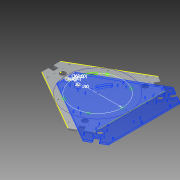
# Autodesk Inventor part: build deck
Saved by Autodesk Inventor 2015 SP1 (Build 190203100, 203)
## iProperties
Created: 2015-01-31
Part Number: build deck
Material: Generic
Document SubType Name: Modeling
Designer: Joseph
Density: 1 g/cm^3
Appearance: Clear
Author: Joseph
Autodesk Inventor part; units mm, degrees
ref_plane "YZ Plane" through (0, 0, 0) normal (1, 0, 0) x (0, 1, 0)
ref_plane "XZ Plane" through (0, 0, 0) normal (0, 1, 0) x (-1, 0, 0)
ref_plane "XY Plane" through (0, 0, 0) normal (0, 0, 1) x (1, 0, 0)
sketch "Sketch1" plane through (0, 0, 0) normal (0, 0, 1) x (1, 0, 0)
  line L0 (-22.3671, -44.8758) -> (185.479, -164.8758)
  line L1 (263.2049, -120.0008) -> (263.2049, 119.9992)
  line L2 (263.2049, 138.0318) -> (240.8188, 150.9564)
  line L3 (201.0957, -173.8921) -> (223.4817, -160.9675)
  line L4 (-37.9837, -10.0104) -> (-37.9837, -35.8596)
  line L5 (263.2049, 138.0318) -> (263.2049, -138.0333)
  line L6 (201.0957, -173.8921) -> (-37.9837, -35.8596)
  line L7 (-37.9837, 9.9896) -> (-17.9837, 9.9896)
  line L8 (-17.9837, 9.9896) -> (-17.9837, -10.0104)
  line L9 (-17.9837, -10.0104) -> (-37.9837, -10.0104)
  line L10 (-37.9837, -35.8596) -> (-37.9837, -10.0104)
  line L11 (-37.9837, 9.9896) -> (-37.9837, 35.8388)
  line L12 (223.49, -160.9627) -> (213.49, -143.6422)
  line L13 (213.49, -143.6422) -> (230.8105, -133.6422)
  line L14 (230.8105, -133.6422) -> (240.8105, -150.9627)
  line L15 (263.2049, -138.0333) -> (240.8105, -150.9627)
  line L16 (223.49, -160.9627) -> (201.0957, -173.8921)
  line L17 (223.5235, 160.9901) -> (213.4873, 143.6905)
  line L18 (213.4873, 143.6905) -> (230.7869, 133.6543)
  line L19 (230.7869, 133.6543) -> (240.7869, 150.9748)
  line L20 (201.1375, 173.9147) -> (223.5235, 160.9901)
  line L21 (240.7869, 150.9748) -> (263.2049, 138.0318)
  line L22 (-37.9837, 35.8388) -> (201.1375, 173.9147)
  point P0 (0, 0)
  dimension "d0" = 20
  dimension "d1" = 20
  dimension "d2" = 20
  dimension "d3" = 20
  dimension "d4" = 20
  dimension "d5" = 20
  constraints: 46 end point, 10 perpendicular, 5 equal length, 5 vertical, 2 collinear, 2 parallel, 1 horizontal, 13 other
  measures "d0" distance of L7.start L7.end
  measures "d1" distance of L7.end L8.end
  measures "d2" distance of L12.start L12.end
  measures "d3" distance of L12.end L13.end
  measures "d4" distance of L17.start L17.end
  measures "d5" distance of L17.end L18.end
extrude "Extrusion1" add sketch "Sketch1" along normal blind 6.35
sketch "Sketch2" plane through (0, 0, 6.35) normal (0, 0, 1) x (1, 0, 0)
  line L0 (201.1375, 173.9147) -> (-37.9837, 35.8388) projected
  line L1 (-37.9837, -35.8596) -> (201.0957, -173.8921) projected
  line L2 (263.2049, -138.0333) -> (263.2049, 138.0318) projected
  line L3 (-13.2714, -20.105) -> (-13.2714, 20.0856) projected
  line L4 (237.2204, -124.5359) -> (202.4143, -144.6312) projected
  line L5 (202.4143, 144.6118) -> (237.2204, 124.5165) projected
  line L6 (-13.2714, -0.0097) -> (263.2049, -0.0008) construction
  line L7 (219.8173, 134.5641) -> (81.556, -104.8758) construction
  line L8 (219.8173, -134.5836) -> (81.5535, 104.8633) construction
  circle A0 centre (142.1099, -0.009) radius 90 construction
  line L9 (-13.2714, -21.259) -> (29.2286, -21.259) construction
  line L10 (29.2286, -21.259) -> (29.2286, 21.241) construction
  line L11 (29.2286, 21.241) -> (-13.2714, 21.241) construction
  line L12 (-13.2714, 21.241) -> (-13.2714, -21.259) construction
  line L13 (-13.2714, -21.259) -> (29.2286, 21.241) construction
  line L14 (29.2286, -21.259) -> (-13.2714, 21.241) construction
  line L15 (-7.5214, -15.509) -> (23.4786, -15.509) construction
  line L16 (23.4786, -15.509) -> (23.4786, 15.491) construction
  line L17 (23.4786, 15.491) -> (-7.5214, 15.491) construction
  line L18 (-7.5214, 15.491) -> (-7.5214, -15.509) construction
  line L19 (-7.5214, -15.509) -> (23.4786, 15.491) construction
  line L20 (23.4786, -15.509) -> (-7.5214, 15.491) construction
  point P0 (0, 0)
  point P1 (7.9786, -0.009)
  point P2 (203.5022, -137.3435)
  point P3 (188.0022, -110.4967)
  point P4 (214.849, -94.9967)
  point P5 (230.349, -121.8435)
  point P6 (230.3489, 121.8255)
  point P7 (214.8489, 94.9787)
  point P8 (188.0021, 110.4787)
  point P9 (203.5021, 137.3255)
  dimension "d8" = 180
  dimension "d9" = 42.5
  dimension "d10" = 42.5
  dimension "d11" = 31
  dimension "d12" = 31
  dimension "d15" = 360
  constraints: 30 end point, 9 midpoint, 5 point on line, 4 coincident, 4 parallel, 3 perpendicular, 2 horizontal, 1 centre point, 13 other
  measures "d8" diameter of A0
  measures "d9" distance of L11.end L10.end
  measures "d10" distance of L10.end L9.end
  measures "d11" distance of L17.end L16.end
  measures "d12" distance of L16.end L15.end
hole "Hole1" at (-7.5214, 15.491, 6.35) at (23.4786, 15.491, 6.35) at (23.4786, -15.509, 6.35) at (-7.5214, -15.509, 6.35) at (230.349, -121.8435, 6.35) at (214.849, -94.9967, 6.35) at (188.0022, -110.4967, 6.35) at (203.5022, -137.3435, 6.35) at (203.5021, 137.3255, 6.35) at (188.0021, 110.4787, 6.35) at (214.8489, 94.9787, 6.35) at (230.3489, 121.8255, 6.35) direction (0, 0, -1) diameter 3.4 end through all clearance for "Socket Head Cap Screw" size "M3" standard "Ansi Metric M Profile"
sketch "Sketch3" plane through (0, 0, 6.35) normal (0, 0, 1) x (1, 0, 0)
  circle A0 centre (23.4786, -15.509) radius 1.7 projected
  circle A1 centre (-7.5214, 15.491) radius 1.7 projected
  line L0 (-17.9837, 9.9896) -> (-17.9837, -10.0104) projected
  line L1 (213.49, -143.6422) -> (230.8105, -133.6422) projected
  line L2 (230.7869, 133.6543) -> (213.4873, 143.6905) projected
  line L3 (-7.5214, 15.491) -> (23.4786, -15.509) construction
  circle A2 centre (7.9786, -0.009) radius 11.25
  circle A3 centre (142.1124, 0.0111) radius 160.0962 construction
  circle A4 centre (209.1968, -116.1422) radius 11.25
  circle A5 centre (209.1619, 116.1844) radius 11.25
  point P0 (0, 0)
  dimension "d24" = 22.5
  dimension "d27" = 360
  constraints: 4 centre point, 3 tangent, 2 end point, 1 midpoint, 7 other
  measures "d24" diameter of A2
extrude "Extrusion2" cut sketch "Sketch3" against normal through all contours A2 | A4 | A5
sketch "Sketch4" plane through (0, 0, 6.35) normal (0, 0, 1) x (1, 0, 0)
  line L0 (201.1375, 173.9147) -> (-37.9837, 35.8388) projected
  line L1 (-37.9837, -35.8596) -> (201.0957, -173.8921) projected
  line L2 (263.2049, -138.0333) -> (263.2049, 138.0318) projected
  circle A0 centre (-13.6913, -49.8848) radius 10 construction
  circle A1 centre (176.8343, -159.8848) radius 10 construction
  line L3 (-8.6913, -41.2245) -> (181.8343, -151.2245) construction
  line L4 (-22.3516, -44.8848) -> (-12.3516, -27.5643) construction
  line L5 (195.4945, -147.5643) -> (185.4945, -164.8848) construction
  circle A2 centre (142.1084, -0.0056) radius 121.0965 construction
  point P0 (0, 0)
  point P1 (86.5715, -96.2245)
  point P2 (253.2049, 0.0075)
  point P3 (253.2049, -109.9925)
  point P4 (253.2049, 110.0075)
  point P5 (86.5488, 96.2003)
  point P6 (181.8115, 151.2003)
  point P7 (-8.714, 41.2003)
  dimension "d31" = 20
  dimension "d32" = 20
  dimension "d35" = 360
  constraints: 3 tangent, 2 coincident, 2 end point, 2 point on line, 1 centre point, 1 midpoint, 1 parallel, 19 other
hole "Hole2" at (86.5715, -96.2245, 6.35) at (-8.6913, -41.2245, 6.35) at (181.8343, -151.2245, 6.35) at (253.2049, -109.9925, 6.35) at (253.2049, 0.0075, 6.35) at (253.2049, 110.0075, 6.35) at (181.8115, 151.2003, 6.35) at (86.5488, 96.2003, 6.35) at (-8.714, 41.2003, 6.35) direction (0, 0, -1) diameter 4.5 end through all clearance for "Socket Head Cap Screw" size "M4" standard "Ansi Metric M Profile"
sketch "Sketch5" plane through (0, 0, 6.35) normal (0, 0, 1) x (1, 0, 0)
  line L0 (201.1375, 173.9147) -> (-37.9837, 35.8388) projected
  line L1 (-37.9837, -35.8596) -> (201.0957, -173.8921) projected
  line L2 (263.2049, -138.0333) -> (263.2049, 138.0318) projected
  circle A0 centre (142.1084, -0.0056) radius 121.0965 construction
  circle A1 centre (142.1084, -0.0056) radius 95 construction
  circle A2 centre (47.0693, 0.6182) radius 12.5 construction
  arc A3 (71.6251, 63.6899) -> (52.1084, 30.4082) centre (142.1084, -0.0056) ccw construction
  arc A4 (67.9155, 67.0423) -> (47.3715, 32.009) centre (142.1084, -0.0056) ccw
  arc A5 (75.3347, 60.3375) -> (56.8452, 28.8075) centre (142.1084, -0.0056) ccw
  arc A6 (75.3347, 60.3375) -> (67.9155, 67.0423) centre (71.6251, 63.6899) ccw
  arc A7 (47.3715, 32.009) -> (56.8452, 28.8075) centre (52.1084, 30.4082) ccw
  circle A8 centre (47.0693, 0.6182) radius 5
  circle A9 centre (94.0486, -81.9999) radius 5
  circle A10 centre (189.0877, -82.6237) radius 5
  circle A11 centre (237.1474, -0.6294) radius 5
  circle A12 centre (190.1681, 81.9888) radius 5
  circle A13 centre (95.129, 82.6126) radius 5
  point P0 (0, 0)
  point P1 (48.0142, 13.0824)
  point P2 (47.8506, -11.8574)
  point P3 (83.7268, -74.9495)
  point P4 (105.2434, -87.5611)
  point P5 (177.8209, -88.0375)
  point P6 (199.5012, -75.7093)
  point P7 (236.2025, -13.0936)
  point P8 (236.3662, 11.8462)
  point P9 (200.49, 74.9383)
  point P10 (178.9733, 87.55)
  point P11 (106.3959, 88.0263)
  point P12 (84.7155, 75.6982)
  dimension "d45" = 190
  dimension "d46" = 25
  dimension "d49" = 360
  dimension "d60" = 10
  dimension "d63" = 360
  constraints: 16 point on circle, 14 centre point, 7 tangent, 1 coincident, 1 concentric, 26 other
  measures "d45" diameter of A1
  measures "d46" diameter of A2
  measures "d60" diameter of A8
extrude "Extrusion3" cut sketch "Sketch5" against normal through all contours A6 A5 A7 A4
hole "Hole3" at (48.0142, 13.0824, 6.35) at (47.8506, -11.8574, 6.35) at (83.7268, -74.9495, 6.35) at (105.2434, -87.5611, 6.35) at (177.8209, -88.0375, 6.35) at (199.5012, -75.7093, 6.35) at (236.2025, -13.0936, 6.35) at (236.3662, 11.8462, 6.35) at (200.49, 74.9383, 6.35) at (178.9733, 87.55, 6.35) at (106.3959, 88.0263, 6.35) at (84.7155, 75.6982, 6.35) direction (0, 0, -1) diameter 3.4 end through all clearance for "Socket Head Cap Screw" size "M3" standard "Ansi Metric M Profile"
extrude "Extrusion4" cut sketch "Sketch5" against normal through all contours A8 | A9 | A10 | A11 | A12 | A13
body "Solid1"
